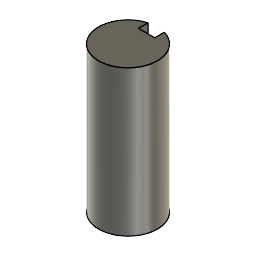
Motor Shaft (Autodesk Fusion 360 design; units mm, degrees)
Autodesk Fusion 360 part; units mm, degrees
sketch "Sketch1" plane through (0, 0, 0) normal (0, 0, 1) x (1, 0, 0)
  circle A0 centre (0, 0) radius 5.45
  line L0 (0, 7.5) -> (0, -6)
  line L1 (-1.5, 5.2395) -> (-1.5, 3.45)
  line L2 (-1.5, 3.45) -> (1.5, 3.45)
  line L3 (1.5, 3.45) -> (1.5, 5.2395)
  circle A1 centre (0, 0) radius 3.2
  line L4 (-2.0805, -2.4314) -> (2.0805, -2.4314)
  point P0 (0, 5.45)
  dimension "d1" = 10.9
  dimension "d2" = 2
  dimension "d3" = 3
  dimension "d4" = 6.4
  dimension "d5" = 4.161
  constraint coincident A0.centre A1.centre
  constraint vertical L0
  constraint coincident A0 L1.start
  constraint parallel L0 L1
  constraint perpendicular L1 L2
  constraint coincident A0 L3.end
  constraint perpendicular L2 L3
  constraint symmetric L0 L1 L3
  constraint coincident A0 P0
  constraint coincident L0 P0
  constraint coincident A0.centre L0
  constraint coincident A1 L4.start
  constraint coincident A1 L4.end
  constraint perpendicular L0 L4
  measures "d1" diameter of A0
  measures "d2" distance of L2 P0
  measures "d3" distance of L1 L3
  measures "d4" diameter of A1
  measures "d5" distance of L4.start L4.end
extrude "Extrude1" add sketch "Sketch1" along normal blind 15
extrude "Extrude2" add sketch "Sketch1" against normal blind 12 contours A0 L0 L2 L3 A1 | A0 L0 L2 L3 | A0 L0 L1 L2 A1 | A0 L0 L1 L2 | L0 A1 L4 | L0 A1 L4 picked at (-0.1505, -2.9331) picked at (0.1505, -2.9331)
extrude "Extrude3" cut sketch "Sketch1" against normal blind 10 from surface at 15 contours A0 L0 L2 L3 | A0 L0 L1 L2
